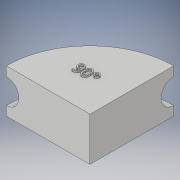
# Autodesk Inventor part: 90deg
Saved by Autodesk Inventor 2017 (Build 210142000, 142)
## iProperties
Created: 2017-01-08
Part Number: 90deg
Material: Generic
Document SubType Name: Modeling
Designer: ICEMAN
Density: 1 g/cm^3
Appearance: Default
Author: ICEMAN
Autodesk Inventor part; units mm, degrees
ref_plane "YZ Plane" through (0, 0, 0) normal (1, 0, 0) x (0, 1, 0)
ref_plane "XZ Plane" through (0, 0, 0) normal (0, 1, 0) x (-1, 0, 0)
ref_plane "XY Plane" through (0, 0, 0) normal (0, 0, 1) x (1, 0, 0)
sketch "Sketch1" plane through (0, 0, 0) normal (0, 1, 0) x (-1, 0, 0)
  line L0 (0, 0) -> (50, 0)
  line L1 (0, 0) -> (0, -50)
  arc A0 (0, -50) -> (50, 0) centre (0, 0) ccw
  dimension "d0" = 50
  dimension "d1" = 50
  dimension "d2" = 50
  constraints: 4 end point, 2 point on circle, 1 centre point, 1 horizontal, 1 perpendicular
  measures "d0" distance of L0.start L0.end
  measures "d1" distance of L0.start L1.end
  measures "d2" radius of A0
extrude "Extrusion1" add sketch "Sketch1" along normal blind 26
sketch "Sketch6" plane through (-50, 0, 0) normal (0, 0, 1) x (1, 0, 0)
  circle A0 centre (-0.0038, 13.0199) radius 7.5
  point P0 (50, 0)
  dimension "d16" = 15
  constraints: 1 centre point
  measures "d16" diameter of A0
sketch3d "3D Sketch1"
  arc A0 (-50, 0, 0) -> (0, 0, -50) centre (0, 0, 0) ccw
  constraints: 3 vertical
sweep "Sweep1" cut profiles "Sketch6" path "3D Sketch1"
sketch "Sketch7" plane through (0, 26, 0) normal (0, 1, 0) x (1, 0, 0)
  line L0 (-28.6018, 23.1431) -> (-22.1569, 23.1431) construction
  line L1 (-22.1569, 23.1431) -> (-22.1569, 20.0191) construction
  line L2 (-22.1569, 20.0191) -> (-28.6018, 20.0191) construction
  line L3 (-28.6018, 20.0191) -> (-28.6018, 23.1431) construction
  spline S0 degree 2 poles (-28.325, 21.0373) (-28.325, 21.5069) (-28.0185, 22.2879) (-27.7516, 22.5697) knots 0 0 0 1 2 2 2
  spline S1 degree 2 poles (-27.7516, 22.5697) (-27.4995, 22.8416) (-26.7629, 23.1431) (-26.3873, 23.1431) knots 0 0 0 1 2 2 2
  spline S2 degree 2 poles (-26.3873, 23.1431) (-25.9671, 23.1431) (-25.2849, 22.8614) (-25.0328, 22.5944) knots 0 0 0 1 2 2 2
  spline S3 degree 2 poles (-25.0328, 22.5944) (-24.7164, 22.2583) (-24.3704, 21.1708) (-24.3704, 20.3353) knots 0 0 0 1 2 2 2
  spline S4 degree 2 poles (-24.3704, 20.3353) (-24.3704, 19.579) (-24.7115, 18.2246) (-25.0427, 17.7747) knots 0 0 0 1 2 2 2
  spline S5 degree 2 poles (-25.0427, 17.7747) (-25.3937, 17.3002) (-26.3823, 16.8009) (-27.104, 16.8009) knots 0 0 0 1 2 2 2
  spline S6 degree 2 poles (-27.104, 16.8009) (-27.2672, 16.8009) (-27.6379, 16.8355) (-27.7961, 16.8849) knots 0 0 0 1 2 2 2
  line L4 (-27.7961, 16.8849) -> (-27.7961, 17.6709)
  line L5 (-27.7961, 17.6709) -> (-27.7565, 17.6709)
  spline S7 degree 2 poles (-27.7565, 17.6709) (-27.6527, 17.6116) (-27.2177, 17.5078) (-26.9953, 17.5078) knots 0 0 0 1 2 2 2
  spline S8 degree 2 poles (-26.9953, 17.5078) (-26.1945, 17.5078) (-25.28, 18.5657) (-25.2157, 19.5444) knots 0 0 0 1 2 2 2
  spline S9 degree 2 poles (-25.2157, 19.5444) (-25.542, 19.322) (-26.1351, 19.1193) (-26.4861, 19.1193) knots 0 0 0 1 2 2 2
  spline S10 degree 2 poles (-26.4861, 19.1193) (-26.8223, 19.1193) (-27.3809, 19.2676) (-27.6626, 19.4802) knots 0 0 0 1 2 2 2
  spline S11 degree 2 poles (-27.6626, 19.4802) (-27.9889, 19.7323) (-28.325, 20.4985) (-28.325, 21.0373) knots 0 0 0 1 2 2 2
  spline S12 degree 2 poles (-25.1959, 20.5183) (-25.1959, 21.1362) (-25.4233, 21.9172) (-25.626, 22.1298) knots 0 0 0 1 2 2 2
  spline S13 degree 2 poles (-25.626, 22.1298) (-25.8039, 22.3275) (-26.1747, 22.4758) (-26.3922, 22.4758) knots 0 0 0 1 2 2 2
  spline S14 degree 2 poles (-26.3922, 22.4758) (-26.8964, 22.4758) (-27.4945, 21.7541) (-27.4945, 21.0719) knots 0 0 0 1 2 2 2
  spline S15 degree 2 poles (-27.4945, 21.0719) (-27.4945, 20.6863) (-27.2968, 20.1871) (-27.0793, 20.0091) knots 0 0 0 1 2 2 2
  spline S16 degree 2 poles (-27.0793, 20.0091) (-26.9211, 19.8806) (-26.5306, 19.7965) (-26.3032, 19.7965) knots 0 0 0 1 2 2 2
  spline S17 degree 2 poles (-26.3032, 19.7965) (-26.0412, 19.7965) (-25.4381, 19.9794) (-25.2108, 20.1327) knots 0 0 0 1 2 2 2
  spline S18 degree 2 poles (-25.2108, 20.1327) (-25.2058, 20.192) (-25.1959, 20.3947) (-25.1959, 20.5183) knots 0 0 0 1 2 2 2
  spline S19 degree 2 poles (-19.783, 19.9695) (-19.783, 18.3284) (-20.7371, 16.791) (-21.7307, 16.791) knots 0 0 0 1 2 2 2
  spline S20 degree 2 poles (-21.7307, 16.791) (-22.7391, 16.791) (-23.6833, 18.358) (-23.6833, 19.9646) knots 0 0 0 1 2 2 2
  spline S21 degree 2 poles (-23.6833, 19.9646) (-23.6833, 21.6157) (-22.7292, 23.1431) (-21.7307, 23.1431) knots 0 0 0 1 2 2 2
  spline S22 degree 2 poles (-21.7307, 23.1431) (-20.7272, 23.1431) (-19.783, 21.5613) (-19.783, 19.9695) knots 0 0 0 1 2 2 2
  spline S23 degree 2 poles (-20.831, 18.1109) (-20.7124, 18.4124) (-20.6135, 19.3418) (-20.6135, 19.9695) knots 0 0 0 1 2 2 2
  spline S24 degree 2 poles (-20.6135, 19.9695) (-20.6135, 20.5973) (-20.7124, 21.5217) (-20.836, 21.8332) knots 0 0 0 1 2 2 2
  spline S25 degree 2 poles (-20.836, 21.8332) (-20.9595, 22.1446) (-21.3896, 22.4659) (-21.7307, 22.4659) knots 0 0 0 1 2 2 2
  spline S26 degree 2 poles (-21.7307, 22.4659) (-22.0718, 22.4659) (-22.5117, 22.1446) (-22.6403, 21.8233) knots 0 0 0 1 2 2 2
  spline S27 degree 2 poles (-22.6403, 21.8233) (-22.7638, 21.5118) (-22.8528, 20.5627) (-22.8528, 19.9646) knots 0 0 0 1 2 2 2
  spline S28 degree 2 poles (-22.8528, 19.9646) (-22.8528, 19.322) (-22.7737, 18.4618) (-22.6452, 18.1257) knots 0 0 0 1 2 2 2
  spline S29 degree 2 poles (-22.6452, 18.1257) (-22.5266, 17.8093) (-22.0866, 17.4683) (-21.7307, 17.4683) knots 0 0 0 1 2 2 2
  spline S30 degree 2 poles (-21.7307, 17.4683) (-21.3945, 17.4683) (-20.9546, 17.7896) (-20.831, 18.1109) knots 0 0 0 1 2 2 2
  spline S31 degree 2 poles (-15.9125, 21.5662) (-15.9125, 20.9088) (-16.8121, 20.0091) (-17.4696, 20.0091) knots 0 0 0 1 2 2 2
  spline S32 degree 2 poles (-17.4696, 20.0091) (-18.1221, 20.0091) (-19.0317, 20.9038) (-19.0317, 21.5662) knots 0 0 0 1 2 2 2
  spline S33 degree 2 poles (-19.0317, 21.5662) (-19.0317, 22.2237) (-18.132, 23.1234) (-17.4696, 23.1234) knots 0 0 0 1 2 2 2
  spline S34 degree 2 poles (-17.4696, 23.1234) (-16.8121, 23.1234) (-15.9125, 22.2237) (-15.9125, 21.5662) knots 0 0 0 1 2 2 2
  spline S35 degree 2 poles (-16.5551, 21.5662) (-16.5551, 21.9617) (-17.0791, 22.5005) (-17.4696, 22.5005) knots 0 0 0 1 2 2 2
  spline S36 degree 2 poles (-17.4696, 22.5005) (-17.8651, 22.5005) (-18.389, 21.9617) (-18.389, 21.5662) knots 0 0 0 1 2 2 2
  spline S37 degree 2 poles (-18.389, 21.5662) (-18.389, 21.1658) (-17.8552, 20.6319) (-17.4696, 20.6319) knots 0 0 0 1 2 2 2
  spline S38 degree 2 poles (-17.4696, 20.6319) (-17.0791, 20.6319) (-16.5551, 21.1757) (-16.5551, 21.5662) knots 0 0 0 1 2 2 2
  point P0 (0, 0)
  constraints: 2 other
extrude "Extrusion4" add sketch "Sketch7" along normal blind 1
body "Solid1"
